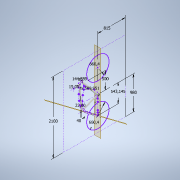
# Autodesk Inventor part: marco_bicicleta
Saved by Autodesk Inventor 2021 (Build 250183000, 183)
## iProperties
Created: 2021-06-19
Part Number: marco_bicicleta
Material: Generic
Document SubType Name: Modeling
Designer: j2seb
Density: 1 g/cm^3
Appearance: Default
Author: j2seb
Autodesk Inventor part; units mm, degrees
ref_plane "YZ Plane" through (0, 0, 0) normal (1, 0, 0) x (0, 1, 0)
ref_plane "XZ Plane" through (0, 0, 0) normal (0, 1, 0) x (-1, 0, 0)
sketch "Sketch1" plane through (0, 0, 0) normal (1, 0, 0) x (0, 1, 0)
  line L0 (-210.4717, 508.276) -> (-4.4381, -1.6752) construction
  line L1 (-4.4381, -1.6752) -> (-4.4381, 508.276) construction
  line L2 (-4.4381, 508.276) -> (-210.4717, 508.276) construction
  line L3 (-984.4381, 1018.8513) -> (1115.5619, 1018.8513) construction
  line L4 (1115.5619, 1018.8513) -> (1115.5619, -816.6752) construction
  line L5 (1115.5619, -816.6752) -> (-984.4381, -816.6752) construction
  line L6 (-984.4381, -816.6752) -> (-984.4381, 1018.8513) construction
  line L7 (-4.4381, -1.6752) -> (-210.4717, 508.276) construction
  spline S0 degree 4 poles (-4.4381, -1.6752) (195.7766, 36.7304) (276.9833, 353.6043) (382.622, 380.7108) (556.0825, 474.2428) knots 0 0 0 0 0 1 1 1 1 1 construction
  spline S1 degree 4 poles (412, 392) (350.8579, 407.6566) (267.6902, 425.3539) (90.9665, 473.8261) (-61.77, 459.9862) (-174.0583, 433.7759) (-273.7121, 378.1254) (-356.4435, 266.3762) (-418.7401, 183.367) (-524.1386, 43.2801) (-547.5831, -1.6752) knots 0 0 0 0 0 0.249566 0.353893 0.455932 0.55166 0.644783 0.741793 1 1 1 1 1 construction
  spline S2 degree 4 poles (537.3261, 544.2428) (496.8844, 552.2205) (277.9738, 570.3179) (51.1685, 574.0588) (-82.5398, 485.8175) (-184.5928, 444.2234) knots 0 0 0 0 0 0.47664 1 1 1 1 1 construction
  spline S3 degree 4 poles (-547.5831, -1.6752) (-453.7397, -1.6752) (-535.4466, -1.6752) (-32.2486, -1.6752) (-137.822, -1.6752) (-4.4381, -1.6752) knots 0 0 0 0 0 0.476897 1 1 1 1 1 construction
  line L8 (560.5514, 457.5648) -> (521.7285, 602.4537)
  line L9 (560.5514, 457.5648) -> (560.5514, 602.4537) construction
  line L10 (560.5514, 602.4537) -> (521.7285, 602.4537) construction
  circle A0 centre (-547.5831, -1.6752) radius 330.2
  circle A1 centre (678.5188, -1.6752) radius 330.2
  line L11 (-210.4717, 508.276) -> (-4.4381, -1.6752)
  line L12 (-4.4381, -1.6752) -> (556.0825, 474.2428)
  line L13 (-547.5831, -1.6752) -> (-4.4381, -1.6752) construction
  line L14 (537.3261, 544.2428) -> (-194.3107, 468.276)
  line L15 (-194.3107, 468.276) -> (-547.5831, -1.6752) construction
  point P0 (0, 0)
  point P1 (169.3986, 120.475)
  point P2 (299.1164, 286.1916)
  point P3 (-177.0425, 425.5356)
  point P4 (322.1858, 413.7845)
  point P5 (197.3229, 441.7976)
  point P6 (49.3376, 463.0025)
  point P7 (-67.9497, 455.482)
  point P8 (-268.5134, 370.7874)
  point P9 (-328.8107, 303.5443)
  point P10 (-385.4046, 227.9635)
  point P11 (-475.6207, 106.1082)
  point P12 (455.4988, 554.1553)
  point P13 (277.1229, 562.4131)
  point P14 (98.4351, 549.1924)
  point P15 (-40, 508.276)
  point P16 (-409.0014, -1.6752)
  point P17 (-196.0454, -1.6752)
  point P18 (-112.8748, -1.6752)
  point P19 (495.5619, 700.109)
  point P20 (498.7461, 727)
  point P21 (-473.3179, -1.6752)
  dimension "d26" = 509.9511
  dimension "d27" = 22
  dimension "d28" = 15
  dimension "d29" = 144.8889
  dimension "d30" = 543.145
  dimension "d31" = 500
  dimension "d32" = 660.4
  dimension "d33" = 660.4
  dimension "d34" = 980
  dimension "d35" = 2100
  dimension "d36" = 815
  dimension "d37" = 70
  dimension "d72" = 40
  constraints: 24 end point, 7 point on line, 6 horizontal alignment, 4 coincident, 3 horizontal, 2 centre point, 2 vertical, 1 collinear, 1 perpendicular, 29 other
  measures "d26" vertical distance of L2.end L1.start
  measures "d27" angle of L1 L0
  measures "d28" angle of L8 L9
  measures "d29" distance of L9.start L9.end
  measures "d30" distance of L1.start point (-547.583, -1.675)
  measures "d31" horizontal distance of L1.start point (495.562, 700.109)
  measures "d32" diameter of A0
  measures "d33" diameter of A1
  measures "d34" horizontal distance of L5.end L1.start
  measures "d35" distance of L4.start L3.start
  measures "d36" vertical distance of L5.end L1.start
  measures "d37" vertical distance of L12.end L14.start
  measures "d72" vertical distance of L14.end L2.end
ref_plane "Work Plane1" through (0, 560.5514, 457.5648) normal (0, -0.258819, 0.9659258) x (1, 0, 0)
sketch "Sketch2" plane through (0, 560.5514, 457.5648) normal (0, -0.258819, 0.9659258) x (1, 0, 0)
  circle A0 centre (0, 0) radius 15
  circle A1 centre (0, 0) radius 12.5
  point P0 (0, -659.8776)
  dimension "d49" = 30
  dimension "d50" = 25
  constraints: 2 centre point, 1 coincident
  measures "d49" diameter of A0
  measures "d50" diameter of A1
extrude "Extrusion1" add sketch "Sketch2" along normal up to surface (150 mm away)
ref_plane "Work Plane3" through (0, -4.4381, -1.6752) normal (0, 0.7622912, 0.6472342) x (-1, 0, 0)
sketch "Sketch3" plane through (0, -4.4381, -1.6752) normal (0, 0.7622912, 0.6472342) x (-1, 0, 0)
  circle A0 centre (0, 0) radius 25
  circle A1 centre (0, 0) radius 22.5
  point P0 (0, -1.5955)
  dimension "d53" = 50
  dimension "d54" = 45
  constraints: 2 centre point, 1 coincident
  measures "d53" diameter of A0
  measures "d54" diameter of A1
extrude "Extrusion2" add sketch "Sketch3" along normal up to surface (735.3104 mm away) separate body
ref_plane "Work Plane4" through (0, -4.4381, -1.6752) normal (0, 0.3746066, -0.9271839) x (-1, 0, 0)
sketch "Sketch4" plane through (0, -4.4381, -1.6752) normal (0, 0.3746066, -0.9271839) x (-1, 0, 0)
  circle A0 centre (0, 0) radius 17.5
  circle A1 centre (0, 0) radius 15
  point P0 (0, 4.7425)
  dimension "d57" = 35
  dimension "d58" = 30
  constraints: 2 centre point, 1 coincident
  measures "d57" diameter of A0
  measures "d58" diameter of A1
extrude "Extrusion3" add sketch "Sketch4" against normal up to surface (550 mm away) separate body
ref_plane "Work Plane5" through (0, 537.3261, 544.2428) normal (0, -0.9946527, -0.1032762) x (1, 0, 0)
sketch "Sketch5" plane through (0, 537.3261, 544.2428) normal (0, -0.9946527, -0.1032762) x (1, 0, 0)
  circle A0 centre (0, 0) radius 20
  circle A1 centre (0, 0) radius 17.5
  point P0 (0, -485.8396)
  dimension "d73" = 40
  dimension "d74" = 35
  constraints: 2 centre point, 1 coincident
  measures "d73" diameter of A0
  measures "d74" diameter of A1
extrude "Extrusion4" add sketch "Sketch5" along normal up to surface (735.5701 mm away) separate body
ref_plane "Work Plane6" through (0, -194.3107, 468.276) normal (0, 0.799339, -0.6008804) x (1, 0, 0)
sketch "Sketch6" plane through (0, -194.3107, 468.276) normal (0, 0.799339, -0.6008804) x (1, 0, 0)
  line L0 (0, 0) -> (-70.1562, 269.3295)
  line L1 (-75, 307.1405) -> (-75, 587.9247)
  line L2 (-17.5, 261.5595) -> (-17.5, -22.2627) projected
  line L3 (0, 257.7247) -> (0, 918.1247) construction
  line L4 (0, 587.9247) -> (-75, 587.9247) construction
  arc A0 (-75, 307.1405) -> (-70.1562, 269.3295) centre (75, 307.1405) ccw
  point P0 (0, 257.5537)
  point P1 (-75, 287.9247)
  dimension "d77" = 75
  dimension "d78" = 300
  dimension "d79" = 150
  constraints: 6 end point, 2 point on circle, 2 point on line, 2 tangent, 1 centre point, 1 coincident, 1 horizontal, 1 parallel
  measures "d77" distance from line of L0.start L1
  measures "d78" distance of point (-75, 287.925) L1.end
  measures "d79" radius of A0
ref_plane "Work Plane7" through (-75, -547.5831, -1.6752) normal (0, -0.6008804, -0.799339) x (1, 0, 0)
sketch "Sketch7" plane through (-75, -547.5831, -1.6752) normal (0, -0.6008804, -0.799339) x (1, 0, 0)
  circle A0 centre (0, 0) radius 10
  circle A1 centre (0, 0) radius 7.5
  point P0 (75, -436.6979)
  dimension "d80" = 20
  dimension "d81" = 15
  constraints: 2 centre point, 1 coincident
  measures "d80" diameter of A0
  measures "d81" diameter of A1
sweep "Sweep1" add profiles "Sketch7" path "Sketch6" separate body path curves L1 A0 L0
mirror "Mirror1" about plane through (0, 0, 0) normal (1, 0, 0) bodies 5 separate body
sketch "Sketch8" plane through (0, 0, 0) normal (1, 0, 0) x (0, 1, 0)
  line L0 (11.7427, -20.7324) -> (-20.619, 17.3821) projected
  circle A0 centre (-4.4381, -1.6752) radius 22.5
  circle A1 centre (-4.4381, -1.6752) radius 20
  point P0 (0, 0)
  dimension "d84" = 45
  dimension "d85" = 40
  constraints: 2 centre point, 1 coincident, 1 midpoint
  measures "d84" diameter of A0
  measures "d85" diameter of A1
extrude "Extrusion5" add sketch "Sketch8" along normal mid plane 75 separate body contours A0 L0 A1 | L0 A1 A0
ref_plane "Work Plane8" through (0, -473.3179, -1.6752) normal (0, 0, 1) x (1, 0, 0)
sketch "Sketch9" plane through (0, -473.3179, -1.6752) normal (0, 0, 1) x (1, 0, 0)
  ellipse E0 centre (0, 468.8798) end of major axis (-17.5, 468.8798) minor radius 16.2257 projected
  ellipse E1 centre (-75, -74.2652) end of major axis (-65, -74.2652) minor radius 7.9934 projected
  line L0 (20, 468.8798) -> (-20, 468.8798) construction
  line L1 (-20, 468.8798) -> (-73.7102, 237.0184)
  line L2 (-75, 225.7348) -> (-75, -74.2652)
  arc A0 (-73.7102, 237.0184) -> (-75, 225.7348) centre (-25, 225.7348) ccw
  point P0 (0, 473.3179)
  dimension "d90" = 40
  dimension "d91" = 50
  dimension "d92" = 300
  constraints: 6 end point, 2 point on circle, 2 tangent, 1 centre point, 1 coincident, 1 horizontal, 1 midpoint, 1 vertical, 1 other
  measures "d90" distance of L0.start L0.end
  measures "d91" radius of A0
  measures "d92" distance of L2.start L2.end
ref_plane "Work Plane9" through (-75, -547.5831, -1.6752) normal (0, -1, 0) x (1, 0, 0)
sketch "Sketch10" plane through (-75, -547.5831, -1.6752) normal (0, -1, 0) x (1, 0, 0)
  circle A0 centre (0, 0) radius 10
  circle A1 centre (0, 0) radius 7.5
  point P0 (75, 1.6752)
  dimension "d93" = 20
  dimension "d94" = 15
  constraints: 2 centre point, 1 coincident
  measures "d93" diameter of A0
  measures "d94" diameter of A1
sweep "Sweep2" add profiles "Sketch10" path "Sketch9" separate body path curves L2 A0 L1
mirror "Mirror2" about plane through (0, 0, 0) normal (1, 0, 0) bodies 8 separate body
sketch "Sketch11" plane through (37.5, -4.4381, -1.6752) normal (1, 0, 0) x (0, 0, -1)
  circle A0 centre (0, 0) radius 22.5 projected
  point P0 (-1.6752, 4.4381)
extrude "Extrusion6" cut sketch "Sketch11" against normal blind 75 bodies 9 8 3 2
ref_plane "Work Plane10" through (0, 48.9223, 43.6312) normal (0, 0.7622912, 0.6472342) x (-1, 0, 0)
body "Solid1"
body "Solid2"
body "Solid3"
body "Solid4"
body "Solid5"
body "Solid6"
body "Solid7"
body "Solid8"
body "Solid9"
